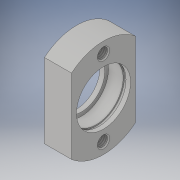
# Autodesk Inventor part: BGTAB6900VV_h
Saved by Autodesk Inventor 2019 (Build 230136000, 136)
## iProperties
Created: 2022-11-21
Part Number: BGTAB6900VV_h
Material: Generic
Catalog Web Link: www.cadenas.de
Description: BGTAB, BGTCA, SBGTA_housing-Bearings with Housings - Space Saving, Small Flange - Retained
Vendor: MISUMI
Document SubType Name: Modeling
Designer: psAdmin
Manufacturer: MISUMI
Mass: 6.24417 g
Surface Area: 36.8237 cm^2
Volume: 6.24417 cm^3
Density: 1 g/cm^3
Appearance: PSOLRGB-175-175-175
Category: PARTsolutions
Company: MISUMI
Title: BGTAB6900VV
Author: Cadenas PARTsolutions
Comments: Bearings with Housings - Space Saving, Small Flange - Retained
PSOL_IDENT_0: {$CADENAS_DATA/23d-libs/misumi/metric/12_bearing_holders/bgtab/housing_bgtab.prj},202 {VTYP=3D},{NB=
PSOL_IDENT_1: BGTAB6900VV_h},{LINA=BGTAB6900VV},{NN=BGTAB, BGTCA, SBGTA_housing},{DATE=25.04.2017 02:57:07},{GEOMD
PSOL_IDENT_2: ATE=10.07.2015 02:13:07},{VERSION=},{LINEID=90},{WBVAR=MATB,ST,SEAL,ALT1},{WBNUMERIC=}  {NB=BGTAB690
PSOL_IDENT_3: 0VV_h},{LINA=BGTAB6900VV},{KT=DUMMY},{PN=BGTAB6900VV},{TYPE=BGTAB},{MATB=S},{MATBALG= 'S' , 'Steel'
PSOL_IDENT_4: , 'SS' , 'Stainless Steel' },{ST=BO},{STALG= 'BO' , 'Black Oxide' , 'ENP' , 'Electroless Nickel Plat
PSOL_IDENT_5: ing' },{BN=6900},{SEAL=VV},{SEALALG= 'ZZ' , 'Double Shielded' , 'VV' , 'Non-Contact Sealed Rubber Se
PSOL_IDENT_6: al' , 'DD' , 'Contact Sealed Rubber Seal' },{DD=10},{D=22},{B=6},{H=40},{W=26},{T=11},{DDHH=19},{A=3
PSOL_IDENT_7: 1},{F=0},{M=M5},{ALT1=},{M3D=5},{MM=1.15},{BDD2=23}
NB: BGTAB6900VV_h
NN: BGTAB, BGTCA, SBGTA_housing
NT: Bearings with Housings - Space Saving, Small Flange - Retained
NBSYN: $PN._h
LINA: BGTAB6900VV
CATALOG: Misumi
PN: BGTAB6900VV
MATB: Steel
ST: Black Oxide
BN: 6900
SEAL: Non-Contact Sealed Rubber Seal
DD: 10
D: 22
B: 6
H: 40
W: 26
T: 11
DDHH: 19
A: 31
F: 0
M: M5
ALT1: Bearing and Retaining Ring Assembled
SUPPLIER: MISUMI
ARTICLENO: BGTAB6900VV_h
BOMINFO: BGTAB6900VV
CREATOR: CADENAS GmbH
Autodesk Inventor part; units mm, degrees
ref_plane "YZ Plane" through (0, 0, 0) normal (1, 0, 0) x (0, 1, 0)
ref_plane "XZ Plane" through (0, 0, 0) normal (0, 1, 0) x (-1, 0, 0)
ref_plane "XY Plane" through (0, 0, 0) normal (0, 0, 1) x (1, 0, 0)
sketch "Sketch_1" plane through (0, 0, 0) normal (1, 0, 0) x (0, 0, -1)
  line L0 (-13, 15.1987) -> (-13, -15.1987)
  arc A0 (-13, -15.1987) -> (13, -15.1987) centre (0, 0) ccw
  line L1 (13, -15.1987) -> (13, 15.1987)
  arc A1 (13, 15.1987) -> (-13, 15.1987) centre (0, 0) ccw
  constraints: 4 end point, 4 point on circle, 2 centre point
extrude "Extrusion1" add sketch "Sketch_1" along normal mid plane 11
sketch "Sketch2" plane through (5.5, 0, 0) normal (1, 0, 0) x (0, 0, -1)
  point P0 (0, 0)
hole "Hole1" at (5.5, 0, 0) direction (-1, 0, 0) diameter 19 depth 11 counterbore diameter 22 counterbore depth 9
sketch "Sketch_9" plane through (0, 0, 0) normal (0, 0, 1) x (1, 0, 0)
  line L0 (3.65, 0) -> (2.5, 0)
  line L1 (2.5, 0) -> (2.5, 11.5)
  line L2 (2.5, 11.5) -> (3.65, 11.5)
  line L3 (3.65, 11.5) -> (3.65, 0)
  line L4 (3.65, 0) -> (2.5, 0)
  constraints: 10 end point
revolve "Revolution1" cut sketch "Sketch_9" angle 360 about axis through (3.65, 0, 0) along (1, 0, 0)
sketch "Sketch_8" plane through (0, 0, 0) normal (0, 0, 1) x (1, 0, 0)
  line L0 (5.5, -15.5) -> (-5.5, -15.5)
  line L1 (-5.5, -15.5) -> (-5.5, -13)
  line L2 (-5.5, -13) -> (-5.067, -13.433)
  line L3 (-5.067, -13.433) -> (5.067, -13.433)
  line L4 (5.067, -13.433) -> (5.5, -13)
  line L5 (5.5, -13) -> (5.5, -15.5)
  line L6 (5.5, -15.5) -> (-5.5, -15.5)
  constraints: 14 end point
revolve "Revolution2" cut sketch "Sketch_8" angle 360 about axis through (5.5, -15.5, 0) along (1, 0, 0)
thread "Thread1" size "M5x0.8" class "6H" standard "ISO Metric profile" full length
sketch "Sketch_2" plane through (0, 0, 0) normal (0, 0, 1) x (1, 0, 0)
  line L0 (5.5, 15.5) -> (-5.5, 15.5)
  line L1 (-5.5, 15.5) -> (-5.5, 18)
  line L2 (-5.5, 18) -> (-5.067, 17.567)
  line L3 (-5.067, 17.567) -> (5.067, 17.567)
  line L4 (5.067, 17.567) -> (5.5, 18)
  line L5 (5.5, 18) -> (5.5, 15.5)
  line L6 (5.5, 15.5) -> (-5.5, 15.5)
  constraints: 14 end point
revolve "Revolution3" cut sketch "Sketch_2" angle 360 about axis through (5.5, 15.5, 0) along (1, 0, 0)
thread "Thread2" size "M5x0.8" class "6H" standard "ISO Metric profile" full length
ref_plane "HOUSING_TO_DUMMY_XY" through (0, 0, 0) normal (0, 0, 1) x (1, 0, 0)
ref_plane "HOUSING_TO_DUMMY_YZ" through (0, 0, 0) normal (1, 0, 0) x (0, 1, 0)
ref_plane "HOUSING_TO_DUMMY_ZX" through (0, 0, 0) normal (0, 1, 0) x (0, 0, 1)
ref_plane "bgcab_to_rring_XY" through (2.5, 0, 0) normal (-1, 0, 0) x (0, 0, -1)
ref_plane "bgcab_to_rring_YZ" through (2.5, 0, 0) normal (0, 0, -1) x (0, -1, 0)
ref_plane "bgcab_to_rring_ZX" through (2.5, 0, 0) normal (0, -1, 0) x (-1, 0, 0)
ref_plane "to_bearings_XY" through (-3.5, 0, 0) normal (-1, 0, 0) x (0, 0, -1)
ref_plane "to_bearings_YZ" through (-3.5, 0, 0) normal (0, 0, -1) x (0, -1, 0)
ref_plane "to_bearings_ZX" through (-3.5, 0, 0) normal (0, -1, 0) x (-1, 0, 0)
body "Solid1"
